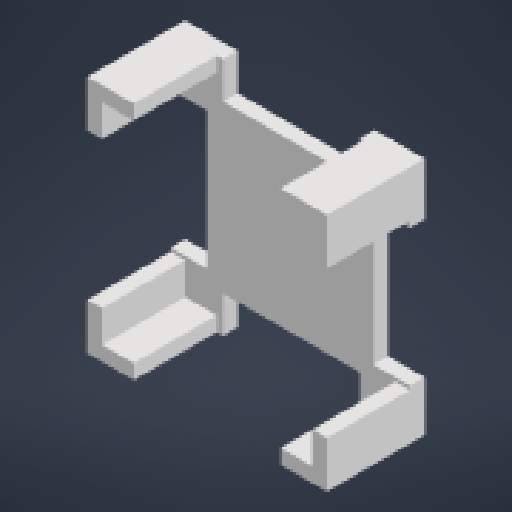
# Autodesk Inventor part: SistemaLiberacion2.2
Saved by Autodesk Inventor 2026.1 (Build 301233000, 233)
## iProperties
Created: 2025-11-13
Part Number: SistemaLiberacion2.2
Material: Genérico
Document SubType Name: Modeling
Designer: usuario
Density: 1 g/cm^3
Appearance: Valor por defecto
Author: usuario
Autodesk Inventor part; units mm, degrees
ref_plane "YZ Plane" through (0, 0, 0) normal (1, 0, 0) x (0, 1, 0)
ref_plane "XZ Plane" through (0, 0, 0) normal (0, 1, 0) x (-1, 0, 0)
ref_plane "XY Plane" through (0, 0, 0) normal (0, 0, 1) x (1, 0, 0)
sketch "Boceto1" plane through (0, 0, 0) normal (0, 0, 1) x (1, 0, 0)
  line L0 (-49, 49) -> (-49, -49)
  line L1 (-49, -49) -> (49, -49)
  line L2 (49, -49) -> (49, 49)
  line L3 (49, 49) -> (-49, 49)
  line L4 (-49, 49) -> (49, -49) construction
  line L5 (-49, -49) -> (49, 49) construction
  line L6 (-43, 43) -> (-43, -43)
  line L7 (-43, -43) -> (43, -43)
  line L8 (43, -43) -> (43, 43)
  line L9 (43, 43) -> (-43, 43)
  line L10 (-43, 43) -> (43, -43) construction
  line L11 (-43, -43) -> (43, 43) construction
  line L12 (-49, -30) -> (49, -30)
  line L13 (-49, 30) -> (49, 30)
  line L14 (-30, -49) -> (-30, 49)
  line L15 (30, -49) -> (30, 49)
  point P0 (0, 0)
  point P1 (0, -30)
  point P2 (0, -49)
  point P3 (-30, 43)
  point P4 (-43, 30)
  point P5 (30, 43)
  point P6 (43, 30)
  point P7 (30, -43)
  point P8 (43, -30)
  point P9 (-30, -43)
  point P10 (-43, -30)
  dimension "d0" = 98
  dimension "d1" = 98
  dimension "d2" = 6
  dimension "d3" = 6
  dimension "d8" = 19
  dimension "d10" = 19
  dimension "d11" = 19
  dimension "d18" = 19
  constraints: 32 end point, 8 point on line, 6 midpoint, 6 perpendicular, 4 parallel, 1 vertical
  measures "d0" distance of L0.start L0.end
  measures "d1" distance of L1.end L0.end
  measures "d2" distance between parallel lines of L1 L7
  measures "d3" distance between parallel lines of L8 L2
  measures "d8" distance of point (0, -30) point (0, -49)
  measures "d10" distance between parallel lines of L14 L0
  measures "d11" distance between parallel lines of L2 L15
  measures "d18" distance between parallel lines of L3 L13
extrude "Extrusión1" add sketch "Boceto1" against normal blind 34 contours L3 L14 L9 L6 L13 L0 | L12 L6 L7 L14 L1 L0 | L3 L2 L13 L8 L9 L15 | L15 L7 L8 L12 L2 L1
sketch "Boceto2" plane through (0, 0, -34) normal (0, 0, -1) x (-1, 0, 0)
  line L0 (49, 49) -> (-49, 49) projected
  line L1 (-49, -49) -> (49, -49) projected
  line L2 (-49, 49) -> (49, 49)
  line L3 (49, 49) -> (49, -49)
  line L4 (49, -49) -> (-49, -49)
  line L5 (-49, -49) -> (-49, 49)
  line L6 (49, -30) -> (43, -30) projected
  line L7 (49, 26) -> (49, -30)
  line L8 (-49, -30) -> (-49, 26)
  line L9 (30, 49) -> (-26, 49)
  line L10 (30, -49) -> (-30, -49)
  line L11 (-28.5, -49) -> (27.5, -49)
  line L12 (27.5, -49) -> (27.5, -34)
  line L13 (27.5, -34) -> (-28.5, -34)
  line L14 (-28.5, -34) -> (-28.5, -49)
  line L15 (-28.5, 34) -> (27.5, 34)
  line L16 (27.5, 34) -> (27.5, 49)
  line L17 (27.5, 49) -> (-28.5, 49)
  line L18 (-28.5, 49) -> (-28.5, 34)
  line L19 (-49, -28.5) -> (-34, -28.5)
  line L20 (-34, -28.5) -> (-34, 27.5)
  line L21 (-34, 27.5) -> (-49, 27.5)
  line L22 (-49, 27.5) -> (-49, -28.5)
  line L23 (34, -28.5) -> (49, -28.5)
  line L24 (49, -28.5) -> (49, 27.5)
  line L25 (49, 27.5) -> (34, 27.5)
  line L26 (34, 27.5) -> (34, -28.5)
  circle A0 centre (0, 0) radius 10.5
  point P0 (-25.1585, 49)
  point P1 (24.6057, -49)
  point P2 (0, 49)
  point P3 (-0.5, 34)
  point P4 (-0.5, -34)
  dimension "d19" = 34
  dimension "d20" = 34
  dimension "d21" = 56
  dimension "d22" = 21.5
  dimension "d23" = 56
  dimension "d24" = 21.5
  dimension "d25" = 56
  dimension "d26" = 34
  dimension "d27" = 34
  dimension "d28" = 21
  constraints: 48 end point, 10 parallel, 7 horizontal, 6 point on line, 5 perpendicular, 4 collinear, 3 midpoint, 1 centre point, 1 coincident
  measures "d19" vertical distance of point (0, 0) point (-0.5, 34)
  measures "d20" vertical distance of point (-0.5, -34) point (0, 0)
  measures "d21" distance between parallel lines of L12 L14
  measures "d22" distance between parallel lines of L3 L12
  measures "d23" distance between parallel lines of L21 L19
  measures "d24" distance between parallel lines of L0 L21
  measures "d25" distance of L25.end L23.start
  measures "d26" distance from line of L26 point (0, 0)
  measures "d27" distance from line of point (0, 0) L20
  measures "d28" diameter of A0
extrude "Extrusión2" add sketch "Boceto2" along normal blind 6 contours L3 L25 L26 L23 L1 L12 L13 L14 L5 L19 L20 L21 L0 L18 L15 L16
sketch "Boceto3" plane through (0, 0, -34) normal (0, 0, 1) x (1, 0, 0)
  line L0 (-13.2963, -27.7616) -> (-27.4385, -13.6195) construction
  line L1 (-27.4385, -13.6195) -> (-16.8319, -3.0129) construction
  line L2 (-2.6897, -17.155) -> (-13.2963, -27.7616) construction
  line L3 (-34, -28.5) -> (-34, 27.5) projected
  line L4 (-34, -10.5) -> (-24.9011, -10.5)
  line L5 (-24.9011, -10.5) -> (-7.2234, -28.1777)
  line L6 (-7.2234, -28.1777) -> (-13.0457, -34)
  line L7 (28.5, -34) -> (-27.5, -34) projected
  line L8 (-34, -10.5) -> (-34, -28.5)
  line L9 (-27.5, -34) -> (-13.0457, -34)
  line L10 (-49, -28.5) -> (-34, -28.5) projected
  line L11 (-34, -28.5) -> (-49, -28.5)
  line L12 (-27.5, -49) -> (-49, -49) projected
  line L13 (-49, -28.5) -> (-49, -49)
  line L14 (-49, -49) -> (-27.5, -49)
  line L15 (-27.5, -49) -> (-27.5, -34)
  line L16 (-13.0457, -34) -> (-27.5, -34)
  circle A0 centre (0, 0) radius 10.5 projected
  line L17 (-49, 49) -> (-27.5, 49) construction
  line L18 (49, -49) -> (28.5, -49) construction
  line L19 (-49, 49) -> (49, -49) construction
  line L20 (49, 49) -> (49, 27.5) construction
  line L21 (-49, -49) -> (49, 49) construction
  line L22 (27.7616, 13.2963) -> (13.6195, 27.4385) construction
  line L23 (13.6195, 27.4385) -> (3.0129, 16.8319) construction
  line L24 (10.5, 34) -> (10.5, 24.9011)
  line L25 (10.5, 24.9011) -> (28.1777, 7.2234)
  line L26 (28.1777, 7.2234) -> (34, 13.0457)
  line L27 (10.5, 34) -> (28.5, 34)
  line L28 (34, 27.5) -> (34, 13.0457)
  line L29 (28.5, 49) -> (28.5, 34)
  line L30 (28.5, 34) -> (28.5, 49)
  line L31 (49, 27.5) -> (49, 49)
  line L32 (28.5, 49) -> (49, 49)
  line L33 (49, 49) -> (49, 27.5)
  line L34 (49, 27.5) -> (34, 27.5)
  line L35 (34, 13.0457) -> (34, 27.5)
  dimension "d29" = 25
  dimension "d30" = 90
  dimension "d31" = 18
  dimension "d41" = 4
  constraints: 52 end point, 10 symmetric about line, 5 collinear, 4 perpendicular, 2 point on line, 1 horizontal
  measures "d29" distance of L4.end L5.end
  measures "d30" angle of L6 L5
  measures "d31" distance from line of L3.start L4
  measures "d41" distance between parallel lines of L5 L0
extrude "Extrusión3" add sketch "Boceto3" along normal blind 2 contours L3 L4 L5 L6 L7 L15 L12 L13 L10 | L27 L29 L32 L31 L34 L28 L26 L25 L24
sketch "Boceto4" plane through (0, 0, -32) normal (0, 0, 1) x (1, 0, 0)
  line L0 (-27.4385, -13.6195) -> (-16.8319, -3.0129) projected
  line L1 (-2.6897, -17.155) -> (-13.2963, -27.7616) projected
  line L2 (-13.2963, -27.7616) -> (-27.4385, -13.6195) projected
  line L3 (-7.2234, -28.1777) -> (-24.9011, -10.5) projected
  line L4 (-13.0457, -34) -> (-7.2234, -28.1777) projected
  line L5 (-10.4679, -24.9332) -> (-7.2234, -28.1777)
  line L6 (28.5, -34) -> (-13.0457, -34) projected
  line L7 (-7.2234, -28.1777) -> (-13.0457, -34)
  line L8 (-24.9011, -10.5) -> (-34, -10.5) projected
  line L9 (-34, -10.5) -> (-34, -28.5) projected
  line L10 (-27.5, -34) -> (-13.0457, -34) projected
  line L11 (-27.5, -49) -> (-27.5, -34) projected
  line L12 (-34, -28.5) -> (-49, -28.5) projected
  line L13 (-49, -49) -> (-30, -49) projected
  line L14 (-49, -30) -> (-49, -49) projected
  line L15 (-49, -28.5) -> (-49, -30) projected
  line L16 (-30, -49) -> (-27.5, -49) projected
  line L17 (30, 49) -> (30, 43) projected
  line L18 (30, 49) -> (28.5, 49) projected
  line L19 (28.5, 49) -> (28.5, 34) projected
  line L20 (28.5, 34) -> (10.5, 34) projected
  line L21 (10.5, 34) -> (10.5, 24.9011) projected
  line L22 (10.5, 24.9011) -> (28.1777, 7.2234) projected
  line L23 (28.1777, 7.2234) -> (34, 13.0457) projected
  line L24 (34, 13.0457) -> (34, 27.5) projected
  line L25 (34, 27.5) -> (49, 27.5) projected
  line L26 (49, 27.5) -> (49, 30) projected
  line L27 (43, 30) -> (49, 30) projected
  line L28 (43, 43) -> (43, 30) projected
  line L29 (30, 43) -> (43, 43) projected
  line L30 (30, 43) -> (43, 43) projected
  line L31 (43, 43) -> (43, 30) projected
  line L32 (43, 30) -> (49, 30) projected
  line L33 (49, 30) -> (49, 49) projected
  line L34 (49, 49) -> (30, 49) projected
  line L35 (30, 49) -> (30, 43) projected
  line L36 (28.227, 13.7617) -> (17.6204, 3.1551) projected
  line L37 (14.0848, 27.9038) -> (28.227, 13.7617) projected
  line L38 (3.4782, 17.2972) -> (14.0848, 27.9038) projected
  point P0 (0, 0)
  point P1 (-24.61, -10.791)
  point P2 (10.791, 24.61)
  point P3 (24.9332, 10.4679)
  constraints: 4 end point, 4 point on line, 1 collinear, 1 perpendicular
extrude "Extrusión4" add sketch "Boceto4" along normal blind 17 contours L2 L1 L3 L4 L10 L11 L16 L13 L14 L15 L12 L9 L8 L0 | L17 L29 L28 L27 L26 L25 L24 L23 L22 L36 L37 L38 L21 L20 L19 L18
